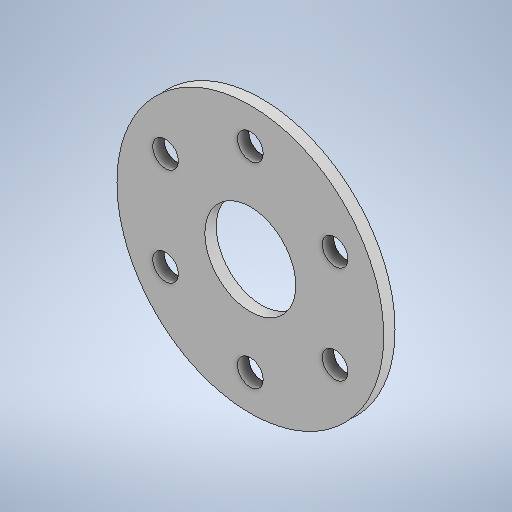
# Autodesk Inventor part: rotor_hub_retainer
Saved by Autodesk Inventor 2025.2 (Build 292293000, 293)
## iProperties
Created: 2025-03-08
Part Number: rotor_hub_retainer
Material: Generic
Document SubType Name: Modeling
Designer: aaron
Density: 1 g/cm^3
Appearance: Default
Author: aaron
Autodesk Inventor part; units mm, degrees
ref_plane "YZ Plane" through (0, 0, 0) normal (1, 0, 0) x (0, 1, 0)
ref_plane "XZ Plane" through (0, 0, 0) normal (0, 1, 0) x (-1, 0, 0)
ref_plane "XY Plane" through (0, 0, 0) normal (0, 0, 1) x (1, 0, 0)
sketch "Sketch1" plane through (0, 0, 0) normal (0, 0, 1) x (1, 0, 0)
  circle A0 centre (0, 0) radius 23.5
  circle A1 centre (0, 0) radius 17.25
  circle A2 centre (0, 17.25) radius 2.25
  circle A3 centre (-14.9389, 8.625) radius 2.25
  circle A4 centre (-14.9389, -8.625) radius 2.25
  circle A5 centre (0, -17.25) radius 2.25
  circle A6 centre (14.9389, -8.625) radius 2.25
  circle A7 centre (14.9389, 8.625) radius 2.25
  circle A8 centre (0, 0) radius 8
  dimension "d1" = 34.5
  dimension "d0" = 47
  dimension "d2" = 4.5
  dimension "d5" = 360
  dimension "d7" = 16
  constraints: 8 centre point, 3 coincident, 1 vertical alignment, 15 other
  measures "d0" diameter of A0
  measures "d2" diameter of A2
  measures "d7" diameter of A8
extrude "Extrusion1" add sketch "Sketch1" along normal blind 2 contours A0 | A1 A6 A5 A4 A3 A2 A7
body "Solid1"
